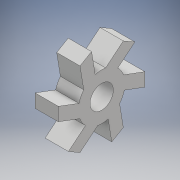
# Autodesk Inventor part: mtv_gear6v2_1-16
Saved by Autodesk Inventor 2018 (Build 220112000, 112)
## iProperties
Created: 2019-01-17
Part Number: mtv_gear6v2_1-16
Material: Generic
Document SubType Name: Modeling
Designer: aditya
Density: 1 g/cm^3
Appearance: Default
Author: aditya
## iProperties of the stored document mtv_gear6v2_1-16_3DPrint.ipt
Created: 2019-01-17
Part Number: mtv_gear6v2_1-16_3DPrint
Material: Generic
Document SubType Name: Modeling
Designer: aditya
Density: 1 g/cm^3
Appearance: Default
Author: aditya
Autodesk Inventor part; units mm, degrees
ref_plane "YZ Plane" through (0, 0, 0) normal (1, 0, 0) x (0, 1, 0)
ref_plane "XZ Plane" through (0, 0, 0) normal (0, 1, 0) x (-1, 0, 0)
ref_plane "XY Plane" through (0, 0, 0) normal (0, 0, 1) x (1, 0, 0)
sketch "Sketch1" plane through (0, 0, 0) normal (1, 0, 0) x (0, 1, 0)
  circle A0 centre (0, 0) radius 1.75
  circle A1 centre (0, 0) radius 3.5
  dimension "d0" = 3.5
  dimension "d1" = 7
  constraints: 2 centre point, 2 coincident
  measures "d0" diameter of A0
  measures "d1" diameter of A1
extrude "Extrusion1" add sketch "Sketch1" along normal blind 3.5
sketch "Sketch2" plane through (3.5, 0, 0) normal (1, 0, 0) x (0, 0, -1)
  circle A0 centre (0, 0) radius 3.5 construction
  line L0 (0, 3.5) -> (0, 2.5) construction
  line L1 (0, 2.5) -> (1.5, 2.5) construction
  line L2 (1.5, 2.5) -> (-1.5, 2.5) construction
  line L3 (0, 3.5) -> (0, 6.5) construction
  line L4 (0, 6.5) -> (-1.5, 2.5)
  line L5 (0, 6.5) -> (2, 6.5)
  line L6 (2, 6.5) -> (0.5, 2.5)
  line L7 (-1.5, 2.5) -> (0.5, 2.5)
  dimension "d4" = 1
  dimension "d5" = 1.5
  dimension "d6" = 3
  dimension "d7" = 3
  dimension "d8" = 2
  constraints: 16 end point, 2 perpendicular, 2 point on line, 2 vertical, 1 collinear, 1 parallel, 1 vertical alignment, 1 other
  measures "d4" distance of L0.start L0.end
  measures "d5" distance of L0.end L1.end
  measures "d6" distance of L1.end L2.end
  measures "d7" distance of L0.start L3.end
  measures "d8" distance of L3.end L5.end
extrude "Extrusion2" add sketch "Sketch2" against normal blind 3.5
pattern_circular "Circular Pattern1" count 6 over 360 about axis through (0, 0, 0) along (1, 0, 0) of "Extrusion2"
body "Solid1"
